Autodesk Fusion 360 part; units mm, degrees
(part 2 of 2)
  spline S276 degree 3 poles (42.600211, -33.226398) (42.604396, -33.231183) (42.608576, -33.235966) (42.612753, -33.240748) (43.093705, -33.791283) (43.530619, -34.323345) (43.918051, -34.838169) knots 0.77492411 0.77492411 0.77492411 0.77492411 0.7768622 0.7768622 0.7768622 1 1 1 1
  spline S277 degree 3 poles (43.918052, -34.838171) (45.010703, -36.290103) (45.798661, -37.579973) (46.316835, -38.956798) (46.437001, -39.276088) (46.541754, -39.597353) (46.632029, -39.919515) knots 0 0 0 0 0.81175235 0.81175235 0.81175235 1 1 1 1
  spline S278 degree 3 poles (46.63203, -39.919519) (46.773514, -40.424429) (46.814784, -40.814498) (46.845813, -41.227728) (46.878851, -41.667711) (46.885019, -42.098557) (46.850272, -42.55527) (46.832546, -42.788246) (46.806855, -43.024869) (46.741299, -43.319536) knots 0 0 0 0 0.38345336 0.38345336 0.38345336 0.79173139 0.79173139 0.79173139 1 1 1 1
  spline S279 degree 3 poles (46.741298, -43.319538) (46.404824, -44.831925) (45.478625, -46.0885) (44.311418, -46.957085) (43.806848, -47.332564) (43.253471, -47.641935) (42.664194, -47.885356) (42.664186, -47.885359) (42.664178, -47.885362) (42.664169, -47.885366) knots 0 0 0 0 0.69818353 0.69818353 0.69818353 1 1 1 1.00000633 1.00000633 1.00000633 1.00000633
  spline S280 degree 3 poles (42.664169, -47.885366) (42.034603, -48.145423) (41.279666, -48.346865) (40.565134, -48.400804) (40.346501, -48.417308) (40.13384, -48.423259) (39.924784, -48.422856) knots 0.00000234 0.00000234 0.00000234 0.00000234 0.76570861 0.76570861 0.76570861 1 1 1 1
  spline S281 degree 3 poles (39.924784, -48.422856) (38.818758, -48.420726) (37.665899, -48.16086) (36.622794, -47.69055) (36.179983, -47.490897) (35.751024, -47.258415) (35.321071, -46.997419) knots 0.00000396 0.00000396 0.00000396 0.00000396 0.70199531 0.70199531 0.70199531 1 1 1 1
  spline S282 degree 3 poles (35.321066, -46.997417) (34.424977, -46.45346) (33.574896, -45.800862) (32.774528, -45.054803) knots 0 0 0 0 0.31676612 0.31676612 0.31676612 0.31676612
extrude "Extrude1" add sketch "Sketch1" against normal blind 2 contours S0 S1 S2 S3 S4 S5 S6 S7 S8 S9 S10 S11 S12 S13 S14 S15 S16 S17 S18 S19 S20 S21 S22 S23 S24 S25 S26 S27 S28 S29 S30 S31 S32 S33 S34 S35 S36 S37 S38 S39 S40 S41 S42 S43 S44 S45 S46 S47 S48 S49 S50 S51 S52 S53 S54 S55 S56 S57 S58 S59 S60 S61 S62 S63 S64 S65 S66 S67 S68 S69 S70 S71 | S194 S195 S196 S197 S198 S199 S200 S201 S202 S203 S204 S205 S206 S207 S208 S209 S210 S211 S212 S213 S214 S215 S216 S217 S218 S219 S220 S221 S222 S223 S224 S225 S226 S227 S228 S229 S230 S231 S232 S233 S234 S235 S236 S237 S238 S239 S240 S241 L6 picked at (21.955896, -33.700003) picked at (39.308943, -18.601274)
extrude "Extrude2" add sketch "Sketch1" along normal blind 5 contours S0 S1 S2 S3 S4 S5 S6 S7 S8 S9 S10 S11 S12 S13 S14 S15 S16 S17 S18 S19 S20 S21 S22 S23 S24 S25 S26 S27 S28 S29 S30 S31 S32 S33 S34 S35 S36 S37 S38 S39 S40 S41 S42 S43 S44 S45 S46 S47 S48 S49 S50 S51 S52 S53 S54 S55 S56 S57 S58 S59 S60 S61 S62 S63 S64 S65 S66 S67 S68 S69 S70 S71 picked at (21.955896, -33.700003)
extrude "Extrude3" add sketch "Sketch1" along normal blind 10 contours S194 S195 S196 S197 S198 S199 S200 S201 S202 S203 S204 S205 S206 S207 S208 S209 S210 S211 S212 S213 S214 S215 S216 S217 S218 S219 S220 S221 S222 S223 S224 S225 S226 S227 S228 S229 S230 S231 S232 S233 S234 S235 S236 S237 S238 S239 S240 S241 L6 picked at (39.308943, -18.601274)
sketch "Sketch2" plane through (0, 0, 10) normal (0, 0, 1) x (-1, 0, 0)
  spline S0 degree 3 poles (-28.777152, 47.61447) (-28.158581, 48.54117) (-27.313864, 49.174865) (-26.365085, 49.423963) knots 0 0 0 0 1 1 1 1
  spline S1 degree 3 poles (-26.365085, 49.423963) (-25.870005, 49.553947) (-24.933082, 49.586358) (-24.398238, 49.491999) knots 0 0 0 0 1 1 1 1
  spline S2 degree 3 poles (-24.398238, 49.491999) (-21.853797, 49.043086) (-20.145962, 46.595318) (-19.808691, 42.913987) knots 0 0 0 0 1 1 1 1
  spline S3 degree 3 poles (-19.808691, 42.913987) (-19.738303, 42.145705) (-19.777142, 40.404034) (-19.883263, 39.569933) knots 0 0 0 0 1 1 1 1
  spline S4 degree 3 poles (-19.883263, 39.569933) (-19.974868, 38.849932) (-20.169101, 37.728624) (-20.298509, 37.172733) knots 0 0 0 0 1 1 1 1
  spline S5 degree 3 poles (-20.298509, 37.172733) (-20.350138, 36.950954) (-20.383684, 36.760803) (-20.373056, 36.750176) knots 0 0 0 0 1 1 1 1
  spline S6 degree 3 poles (-20.373056, 36.750176) (-20.362429, 36.739548) (-20.207496, 36.975057) (-20.02876, 37.273529) knots 0 0 0 0 1 1 1 1
  spline S7 degree 3 poles (-20.02876, 37.273529) (-18.11849, 40.463515) (-15.8391, 43.11864) (-13.903666, 44.40829) knots 0 0 0 0 1 1 1 1
  spline S8 degree 3 poles (-13.903666, 44.40829) (-13.13197, 44.9225) (-12.4509, 45.23528) (-11.669465, 45.434349) knots 0 0 0 0 1 1 1 1
  spline S9 degree 3 poles (-11.669465, 45.434349) (-11.12034, 45.574233) (-10.211189, 45.587693) (-9.705467, 45.463417) knots 0 0 0 0 1 1 1 1
  spline S10 degree 3 poles (-9.705467, 45.463417) (-8.958562, 45.27987) (-8.179688, 44.834118) (-7.596024, 44.256169) knots 0 0 0 0 1 1 1 1
  spline S11 degree 3 poles (-7.596024, 44.256169) (-6.902032, 43.568975) (-6.551135, 42.561718) (-6.474, 41.035376) knots 0 0 0 0 1 1 1 1
  spline S12 degree 3 poles (-6.474, 41.035376) (-6.338825, 38.360532) (-7.582333, 35.682392) (-10.063361, 33.304973) knots 0 0 0 0 1 1 1 1
  spline S13 degree 3 poles (-10.063361, 33.304973) (-10.912309, 32.49148) (-11.717344, 31.841911) (-12.942719, 30.981678) knots 0 0 0 0 1 1 1 1
  spline S14 degree 3 poles (-12.942719, 30.981678) (-13.486476, 30.599953) (-14.664879, 29.844231) (-14.781144, 29.80268) knots 0 0 0 0 1 1 1 1
  spline S15 degree 3 poles (-14.781144, 29.80268) (-14.813838, 29.790993) (-14.829778, 29.770067) (-14.816565, 29.756169) knots 0 0 0 0 1 1 1 1
  spline S16 degree 3 poles (-14.816565, 29.756169) (-14.803352, 29.742275) (-14.554706, 29.781213) (-14.264021, 29.842704) knots 0 0 0 0 1 1 1 1
  spline S17 degree 3 poles (-14.264021, 29.842704) (-13.428167, 30.019514) (-12.387035, 30.189924) (-11.439225, 30.305062) knots 0 0 0 0 1 1 1 1
  spline S18 degree 3 poles (-11.439225, 30.305062) (-10.694335, 30.39555) (-10.318137, 30.411456) (-8.906743, 30.412145) knots 0 0 0 0 1 1 1 1
  spline S19 degree 3 poles (-8.906743, 30.412145) (-7.429716, 30.412867) (-7.176998, 30.401447) (-6.587244, 30.307359) knots 0 0 0 0 1 1 1 1
  spline S20 degree 3 poles (-6.587244, 30.307359) (-4.61966, 29.993447) (-3.257425, 29.398503) (-2.302777, 28.436158) knots 0 0 0 0 1 1 1 1
  spline S21 degree 3 poles (-2.302777, 28.436158) (-1.404569, 27.53071) (-0.964594, 26.480042) (-0.898892, 25.083663) knots 0 0 0 0 1 1 1 1
  spline S22 degree 3 poles (-0.898892, 25.083663) (-0.752423, 21.97074) (-2.495588, 19.901678) (-5.951833, 19.086041) knots 0 0 0 0 1 1 1 1
  spline S23 degree 3 poles (-5.951833, 19.086041) (-8.285184, 18.535394) (-11.801198, 18.57942) (-15.197135, 19.201807) knots 0 0 0 0 1 1 1 1
  spline S24 degree 3 poles (-15.197135, 19.201807) (-15.472515, 19.252277) (-15.706188, 19.285206) (-15.71641, 19.274984) knots 0 0 0 0 1 1 1 1
  spline S25 degree 3 poles (-15.71641, 19.274984) (-15.726633, 19.264761) (-15.663483, 19.206281) (-15.576077, 19.145026) knots 0 0 0 0 1 1 1 1
  spline S26 degree 3 poles (-15.576077, 19.145026) (-15.173173, 18.862672) (-14.403009, 18.229035) (-13.855618, 17.729554) knots 0 0 0 0 1 1 1 1
  spline S27 degree 3 poles (-13.855618, 17.729554) (-11.319411, 15.415325) (-9.535422, 12.521165) (-8.985416, 9.828637) knots 0 0 0 0 1 1 1 1
  spline S28 degree 3 poles (-8.985416, 9.828637) (-8.541535, 7.655641) (-8.849932, 5.515577) (-9.799961, 4.176243) knots 0 0 0 0 1 1 1 1
  spline S29 degree 3 poles (-9.799961, 4.176243) (-10.248531, 3.543857) (-11.043643, 3.01215) (-11.885678, 2.781482) knots 0 0 0 0 1 1 1 1
  spline S30 degree 3 poles (-11.885678, 2.781482) (-12.362987, 2.650728) (-13.37267, 2.662599) (-13.879642, 2.804928) knots 0 0 0 0 1 1 1 1
  spline S31 degree 3 poles (-13.879642, 2.804928) (-16.035873, 3.410271) (-18.317612, 5.96279) (-20.405058, 10.10473) knots 0 0 0 0 1 1 1 1
  spline S32 degree 3 poles (-20.405058, 10.10473) (-20.621428, 10.534053) (-20.809268, 10.885434) (-20.822481, 10.885577) knots 0 0 0 0 1 1 1 1
  spline S33 degree 3 poles (-20.822481, 10.885577) (-20.835694, 10.88572) (-20.839472, 10.577696) (-20.830878, 10.201083) knots 0 0 0 0 1 1 1 1
  spline S34 degree 3 poles (-20.830878, 10.201083) (-20.800341, 8.862913) (-20.965717, 7.099114) (-21.2307, 5.936803) knots 0 0 0 0 1 1 1 1
  spline S35 degree 3 poles (-21.2307, 5.936803) (-21.953131, 2.767962) (-23.46365, 0.994904) (-25.819403, 0.550548) knots 0 0 0 0 1 1 1 1
  spline S36 degree 3 poles (-25.819403, 0.550548) (-26.276354, 0.464355) (-27.303759, 0.478399) (-27.762296, 0.577105) knots 0 0 0 0 1 1 1 1
  spline S37 degree 3 poles (-27.762296, 0.577105) (-29.380756, 0.925504) (-30.471677, 2.110585) (-30.979854, 4.072385) knots 0 0 0 0 1 1 1 1
  spline S38 degree 3 poles (-30.979854, 4.072385) (-31.228572, 5.032546) (-31.272789, 5.499233) (-31.272596, 7.162009) knots 0 0 0 0 1 1 1 1
  spline S39 degree 3 poles (-31.272596, 7.162009) (-31.272402, 8.704189) (-31.219619, 9.467197) (-31.030104, 10.666355) knots 0 0 0 0 1 1 1 1
  spline S40 degree 3 poles (-31.030104, 10.666355) (-30.971872, 11.03482) (-30.969098, 11.198786) (-31.022394, 11.12191) knots 0 0 0 0 1 1 1 1
  spline S41 degree 3 poles (-31.022394, 11.12191) (-31.030028, 11.1109) (-31.140908, 10.92892) (-31.268795, 10.717512) knots 0 0 0 0 1 1 1 1
  spline S42 degree 3 poles (-31.268795, 10.717512) (-32.09923, 9.344737) (-33.682992, 7.788682) (-35.140585, 6.913456) knots 0 0 0 0 1 1 1 1
  spline S43 degree 3 poles (-35.140585, 6.913456) (-36.521936, 6.084012) (-37.649445, 5.70804) (-38.888276, 5.663775) knots 0 0 0 0 1 1 1 1
  spline S44 degree 3 poles (-38.888276, 5.663775) (-39.709456, 5.634433) (-40.245182, 5.722796) (-40.924003, 5.999548) knots 0 0 0 0 1 1 1 1
  spline S45 degree 3 poles (-40.924003, 5.999548) (-42.412514, 6.606408) (-43.266225, 7.780936) (-43.456796, 9.48414) knots 0 0 0 0 1 1 1 1
  spline S46 degree 3 poles (-43.456796, 9.48414) (-43.616225, 10.909023) (-42.996088, 13.033743) (-41.979428, 14.545917) knots 0 0 0 0 1 1 1 1
  spline S47 degree 3 poles (-41.979428, 14.545917) (-41.293675, 15.565904) (-40.264162, 16.673275) (-39.248628, 17.483241) knots 0 0 0 0 1 1 1 1
  spline S48 degree 3 poles (-39.248628, 17.483241) (-38.697195, 17.92305) (-37.559702, 18.70613) (-37.002416, 19.02959) knots 0 0 0 0 1 1 1 1
  spline S49 degree 3 poles (-37.002416, 19.02959) (-36.824039, 19.133123) (-36.678096, 19.236237) (-36.678096, 19.258731) knots 0 0 0 0 1 1 1 1
  spline S50 degree 3 poles (-36.678096, 19.258731) (-36.678096, 19.281227) (-36.695612, 19.288805) (-36.717023, 19.275573) knots 0 0 0 0 1 1 1 1
  spline S51 degree 3 poles (-36.717023, 19.275573) (-36.738434, 19.262341) (-37.173133, 19.217823) (-37.68302, 19.176643) knots 0 0 0 0 1 1 1 1
  spline S52 degree 3 poles (-37.68302, 19.176643) (-42.00013, 18.827983) (-45.508277, 19.629245) (-47.812293, 21.490171) knots 0 0 0 0 1 1 1 1
  spline S53 degree 3 poles (-47.812293, 21.490171) (-48.837616, 22.318308) (-49.53917, 23.300587) (-49.803184, 24.277686) knots 0 0 0 0 1 1 1 1
  spline S54 degree 3 poles (-49.803184, 24.277686) (-49.942622, 24.793725) (-49.943332, 25.611328) (-49.80482, 26.123575) knots 0 0 0 0 1 1 1 1
  spline S55 degree 3 poles (-49.80482, 26.123575) (-49.3646, 27.751308) (-47.772047, 29.18037) (-45.585744, 29.909516) knots 0 0 0 0 1 1 1 1
  spline S56 degree 3 poles (-45.585744, 29.909516) (-44.371551, 30.314458) (-43.211242, 30.465773) (-41.609147, 30.428102) knots 0 0 0 0 1 1 1 1
  spline S57 degree 3 poles (-41.609147, 30.428102) (-40.042242, 30.391257) (-38.585558, 30.162583) (-36.798241, 29.672875) knots 0 0 0 0 1 1 1 1
  spline S58 degree 3 poles (-36.798241, 29.672875) (-36.104288, 29.482739) (-34.502045, 28.970831) (-34.011496, 28.782527) knots 0 0 0 0 1 1 1 1
  spline S59 degree 3 poles (-34.011496, 28.782527) (-33.926302, 28.749826) (-33.923577, 28.753712) (-33.987472, 28.816798) knots 0 0 0 0 1 1 1 1
  spline S60 degree 3 poles (-33.987472, 28.816798) (-34.027112, 28.855936) (-34.286566, 29.080518) (-34.56404, 29.315872) knots 0 0 0 0 1 1 1 1
  spline S61 degree 3 poles (-34.56404, 29.315872) (-37.459824, 31.772092) (-40.176255, 34.522567) (-41.680793, 36.521819) knots 0 0 0 0 1 1 1 1
  spline S62 degree 3 poles (-41.680793, 36.521819) (-42.91714, 38.164698) (-43.5687, 39.364673) (-43.935882, 40.675021) knots 0 0 0 0 1 1 1 1
  spline S63 degree 3 poles (-43.935882, 40.675021) (-44.082376, 41.197812) (-44.118476, 42.215448) (-44.008123, 42.711464) knots 0 0 0 0 1 1 1 1
  spline S64 degree 3 poles (-44.008123, 42.711464) (-43.761857, 43.818382) (-42.875081, 44.768754) (-41.595179, 45.297459) knots 0 0 0 0 1 1 1 1
  spline S65 degree 3 poles (-41.595179, 45.297459) (-41.00791, 45.540045) (-40.577769, 45.62411) (-39.930185, 45.622861) knots 0 0 0 0 1 1 1 1
  spline S66 degree 3 poles (-39.930185, 45.622861) (-38.88069, 45.620843) (-37.959139, 45.323304) (-36.774015, 44.603896) knots 0 0 0 0 1 1 1 1
  spline S67 degree 3 poles (-36.774015, 44.603896) (-34.502488, 43.225002) (-32.467553, 40.903967) (-30.578279, 37.537086) knots 0 0 0 0 1 1 1 1
  spline S68 degree 3 poles (-30.578279, 37.537086) (-30.492135, 37.383568) (-30.414524, 37.265095) (-30.405808, 37.273811) knots 0 0 0 0 1 1 1 1
  spline S69 degree 3 poles (-30.405808, 37.273811) (-30.397093, 37.282526) (-30.409562, 37.559482) (-30.433518, 37.889264) knots 0 0 0 0 1 1 1 1
  spline S70 degree 3 poles (-30.433518, 37.889264) (-30.457475, 38.219047) (-30.477736, 39.033089) (-30.478545, 39.698245) knots 0 0 0 0 1 1 1 1
  spline S71 degree 3 poles (-30.478545, 39.698245) (-30.482926, 43.298639) (-29.92491, 45.894977) (-28.777152, 47.61447) knots 0 0 0 0 1 1 1 1
  spline S72 degree 3 poles (-32.472573, 7.085931) (-32.472337, 6.758703) (-32.47025, 6.47465) (-32.464816, 6.218515) (-32.443264, 5.202689) (-32.348926, 4.572177) (-32.141514, 3.771474) knots -0.98475985 -0.98475985 -0.98475985 -0.98475985 -0.78645882 -0.78645882 -0.78645882 -0.00000048 -0.00000048 -0.00000048 -0.00000048
  spline S73 degree 3 poles (-32.141514, 3.771474) (-31.941823, 3.000576) (-31.656083, 2.30244) (-31.269202, 1.691236) (-30.525995, 0.5171) (-29.367827, -0.304768) (-28.01483, -0.596021) knots -1 -1 -1 -1 -0.65765407 -0.65765407 -0.65765407 0 0 0 0
  spline S74 degree 3 poles (-28.014829, -0.596022) (-27.950904, -0.609782) (-27.889104, -0.620859) (-27.827195, -0.63056) (-27.463404, -0.687562) (-27.071573, -0.706087) (-26.675131, -0.706342) (-26.298777, -0.706584) (-25.956294, -0.696435) (-25.596974, -0.628658) knots -1 -1 -1 -1 -0.91970835 -0.91970835 -0.91970835 -0.44790095 -0.44790095 -0.44790095 0 0 0 0
  spline S75 degree 3 poles (-25.596974, -0.628658) (-24.497154, -0.421203) (-23.49334, 0.049053) (-22.668932, 0.765695) (-21.368047, 1.896529) (-20.539039, 3.57199) (-20.060719, 5.670071) knots -1 -1 -1 -1 -0.61209687 -0.61209687 -0.61209687 0 0 0 0
  spline S76 degree 3 poles (-20.060719, 5.670071) (-19.98592, 5.998167) (-19.921486, 6.352401) (-19.865458, 6.727006) knots -1 -1 -1 -1 -0.75017991 -0.75017991 -0.75017991 -0.75017991
  spline S77 degree 3 poles (-19.865458, 6.727006) (-19.506115, 6.170373) (-19.141135, 5.65369) (-18.770183, 5.177884) (-17.363844, 3.374033) (-15.876078, 2.119017) (-14.203993, 1.649594) knots -0.7575867 -0.7575867 -0.7575867 -0.7575867 -0.59946487 -0.59946487 -0.59946487 -0.00000016 -0.00000016 -0.00000016 -0.00000016
  spline S78 degree 3 poles (-14.203993, 1.649594) (-14.154601, 1.635728) (-14.106084, 1.623554) (-14.057883, 1.612546) (-13.622212, 1.513049) (-13.179919, 1.486531) (-12.731334, 1.490683) (-12.335824, 1.494343) (-11.971813, 1.513674) (-11.568631, 1.624122) knots -1 -1 -1 -1 -0.94446886 -0.94446886 -0.94446886 -0.44254044 -0.44254044 -0.44254044 0 0 0 0
  spline S79 degree 3 poles (-11.56863, 1.624122) (-11.508701, 1.640539) (-11.449191, 1.658047) (-11.39012, 1.676601) (-10.355489, 2.00156) (-9.438052, 2.612334) (-8.821191, 3.481973) knots -1 -1 -1 -1 -0.9459899 -0.9459899 -0.9459899 0 0 0 0
  spline S80 degree 3 poles (-8.821191, 3.481973) (-8.647751, 3.726486) (-8.494712, 3.986098) (-8.360502, 4.257492) (-7.544378, 5.907835) (-7.383214, 7.980989) (-7.809695, 10.068803) knots -1 -1 -1 -1 -0.85877638 -0.85877638 -0.85877638 -0.00000001 -0.00000001 -0.00000001 -0.00000001
  spline S81 degree 3 poles (-7.809695, 10.068803) (-8.344019, 12.684563) (-9.857007, 15.321979) (-11.995177, 17.583099) knots -1 -1 -1 -1 -0.135529 -0.135529 -0.135529 -0.135529
  spline S82 degree 3 poles (-11.995177, 17.583099) (-9.651698, 17.410094) (-7.441319, 17.501575) (-5.676216, 17.918121) knots -0.67640459 -0.67640459 -0.67640459 -0.67640459 -0.00000003 -0.00000003 -0.00000003 -0.00000003
  spline S83 degree 3 poles (-5.676216, 17.918121) (-3.741213, 18.374762) (-2.16329, 19.223358) (-1.107088, 20.50976) (-0.083649, 21.756259) (0.382779, 23.376118) (0.299782, 25.140063) knots -1 -1 -1 -1 -0.49212315 -0.49212315 -0.49212315 -0.00000001 -0.00000001 -0.00000001 -0.00000001
  spline S84 degree 3 poles (0.299782, 25.140063) (0.288429, 25.381356) (0.267255, 25.617741) (0.235266, 25.849544) (0.052564, 27.173435) (-0.525731, 28.348698) (-1.450848, 29.281272) knots -1 -1 -1 -1 -0.85099689 -0.85099689 -0.85099689 -0.00000029 -0.00000029 -0.00000029 -0.00000029
  spline S85 degree 3 poles (-1.450848, 29.281272) (-1.547282, 29.378484) (-1.647099, 29.472688) (-1.750221, 29.563762) (-2.911566, 30.58943) (-4.455271, 31.182396) (-6.398185, 31.492372) knots -1 -1 -1 -1 -0.91844647 -0.91844647 -0.91844647 0 0 0 0
  spline S86 degree 3 poles (-6.398188, 31.492372) (-6.5613, 31.518395) (-6.714675, 31.54079) (-6.878045, 31.558344) (-7.343172, 31.608321) (-7.809609, 31.612681) (-8.907329, 31.612145) knots -1 -1 -1 -1 -0.7400635 -0.7400635 -0.7400635 -0.00000004 -0.00000004 -0.00000004 -0.00000004
  spline S87 degree 3 poles (-8.907329, 31.612145) (-9.081721, 31.61206) (-9.240949, 31.611744) (-9.387832, 31.611081) (-9.687499, 31.609728) (-9.933711, 31.607004) (-10.15681, 31.601569) knots -1 -1 -1 -1 -0.87721557 -0.87721557 -0.87721557 -0.62671458 -0.62671458 -0.62671458 -0.62671458
  spline S88 degree 3 poles (-10.15681, 31.601569) (-9.84093, 31.871196) (-9.537673, 32.14671) (-9.233118, 32.438546) knots -0.34136527 -0.34136527 -0.34136527 -0.34136527 0 0 0 0
  spline S89 degree 3 poles (-9.233117, 32.438547) (-8.974453, 32.686409) (-8.727402, 32.938203) (-8.492197, 33.193771) (-6.307323, 35.5678) (-5.134749, 38.310175) (-5.275529, 41.095942) knots -1 -1 -1 -1 -0.90281087 -0.90281087 -0.90281087 0 0 0 0
  spline S90 degree 3 poles (-5.275529, 41.095942) (-5.29661, 41.513089) (-5.336609, 41.90565) (-5.399734, 42.278186) (-5.591289, 43.408642) (-6.024456, 44.38876) (-6.751681, 45.108861) knots -1 -1 -1 -1 -0.7521372 -0.7521372 -0.7521372 -0.00000071 -0.00000071 -0.00000071 -0.00000071
  spline S91 degree 3 poles (-6.751681, 45.108861) (-7.495413, 45.845312) (-8.422699, 46.383888) (-9.419095, 46.628745) knots -1 -1 -1 -1 0 0 0 0
  spline S92 degree 3 poles (-9.419098, 46.628746) (-9.682541, 46.693485) (-9.93614, 46.722202) (-10.200068, 46.73762) (-10.786586, 46.771883) (-11.387538, 46.74449) (-11.965692, 46.597212) knots -1 -1 -1 -1 -0.68965977 -0.68965977 -0.68965977 0 0 0 0
  spline S93 degree 3 poles (-11.965701, 46.597209) (-12.87689, 46.365086) (-13.713118, 45.977261) (-14.569077, 45.406903) knots -1 -1 -1 -1 -0.00000026 -0.00000026 -0.00000026 -0.00000026
  spline S94 degree 3 poles (-14.569077, 45.406903) (-14.911886, 45.178477) (-15.254546, 44.919092) (-15.598078, 44.631736) (-16.591639, 43.800646) (-17.596183, 42.734487) (-18.575476, 41.49903) knots -1 -1 -1 -1 -0.84460942 -0.84460942 -0.84460942 -0.39518925 -0.39518925 -0.39518925 -0.39518925
  spline S95 degree 3 poles (-18.575476, 41.49903) (-18.567986, 42.065666) (-18.574975, 42.600839) (-18.613695, 43.023469) knots -0.43466848 -0.43466848 -0.43466848 -0.43466848 -0.00000013 -0.00000013 -0.00000013 -0.00000013
  spline S96 degree 3 poles (-18.613695, 43.023469) (-18.792964, 44.980199) (-19.328589, 46.680005) (-20.231405, 48.014131) (-21.174019, 49.407066) (-22.560867, 50.386367) (-24.189744, 50.673748) knots -1 -1 -1 -1 -0.51078259 -0.51078259 -0.51078259 0 0 0 0
  spline S97 degree 3 poles (-24.189751, 50.673749) (-24.546559, 50.736698) (-24.905035, 50.750906) (-25.276254, 50.745394) (-25.755317, 50.73828) (-26.214933, 50.704056) (-26.669813, 50.584627) knots -1 -1 -1 -1 -0.56341737 -0.56341737 -0.56341737 -0.0000016 -0.0000016 -0.0000016 -0.0000016
  spline S98 degree 3 poles (-26.669813, 50.584627) (-27.932868, 50.253016) (-29.016834, 49.416859) (-29.775229, 48.280685) knots -1 -1 -1 -1 0 0 0 0
  spline S99 degree 3 poles (-29.77523, 48.280684) (-29.847265, 48.172766) (-29.917006, 48.062423) (-29.984476, 47.949714) (-30.98906, 46.27158) (-31.494286, 44.103071) (-31.637272, 41.383046) knots -1 -1 -1 -1 -0.94694366 -0.94694366 -0.94694366 -0.15697726 -0.15697726 -0.15697726 -0.15697726
  spline S100 degree 3 poles (-31.637272, 41.383046) (-33.018363, 43.215897) (-34.509624, 44.633123) (-36.151323, 45.629691) knots -0.65396261 -0.65396261 -0.65396261 -0.65396261 0 0 0 0
  spline S101 degree 3 poles (-36.151325, 45.629692) (-36.316378, 45.729885) (-36.478865, 45.82388) (-36.63982, 45.911774) (-37.742242, 46.513782) (-38.815354, 46.820718) (-39.92787, 46.822859) knots -1 -1 -1 -1 -0.87259897 -0.87259897 -0.87259897 -0.0000021 -0.0000021 -0.0000021 -0.0000021
  spline S102 degree 3 poles (-39.92787, 46.822859) (-40.680329, 46.82431) (-41.365365, 46.690737) (-42.05332, 46.406561) knots -1 -1 -1 -1 0 0 0 0
  spline S103 degree 3 poles (-42.053328, 46.406558) (-42.161651, 46.361811) (-42.268086, 46.314431) (-42.372532, 46.264469) (-43.780089, 45.591165) (-44.856208, 44.42513) (-45.179484, 42.972067) knots -1 -1 -1 -1 -0.93092246 -0.93092246 -0.93092246 0 0 0 0
  spline S104 degree 3 poles (-45.179484, 42.972066) (-45.269477, 42.567564) (-45.279189, 42.190068) (-45.270967, 41.782869) (-45.261103, 41.294339) (-45.223275, 40.821945) (-45.091374, 40.351235) knots -1 -1 -1 -1 -0.54539945 -0.54539945 -0.54539945 0 0 0 0
  spline S105 degree 3 poles (-45.091374, 40.351233) (-44.676032, 38.869017) (-43.922977, 37.505603) (-42.639618, 35.800255) knots -1 -1 -1 -1 0 0 0 0
  spline S106 degree 3 poles (-42.639617, 35.800255) (-41.642718, 34.475561) (-40.206304, 32.912548) (-38.553365, 31.312101) knots -1 -1 -1 -1 -0.37843695 -0.37843695 -0.37843695 -0.37843695
  spline S107 degree 3 poles (-38.553365, 31.312101) (-39.584175, 31.503217) (-40.567212, 31.603933) (-41.580937, 31.62777) knots -0.60844734 -0.60844734 -0.60844734 -0.60844734 0 0 0 0
  spline S108 degree 3 poles (-41.580938, 31.62777) (-43.272142, 31.667537) (-44.618653, 31.497025) (-45.965395, 31.047877) knots -1 -1 -1 -1 -0.00000011 -0.00000011 -0.00000011 -0.00000011
  spline S109 degree 3 poles (-45.965395, 31.047877) (-46.561441, 30.849092) (-47.122818, 30.602856) (-47.641897, 30.314192) (-49.271077, 29.40819) (-50.519992, 28.075651) (-50.963204, 26.436861) (-50.963206, 26.436851) (-50.963209, 26.436842) (-50.963211, 26.436833) knots -1 -1 -1 -1 -0.75837207 -0.75837207 -0.75837207 0 0 0 0.00000564 0.00000564 0.00000564 0.00000564
  spline S110 degree 3 poles (-50.963211, 26.436833) (-50.963214, 26.436824) (-50.963216, 26.436815) (-50.963219, 26.436805) (-51.02331, 26.214573) (-51.058271, 25.996182) (-51.080545, 25.773981) (-51.140844, 25.172463) (-51.124068, 24.565794) (-50.96164, 23.964669) knots -1.00001792 -1.00001792 -1.00001792 -1.00001792 -1 -1 -1 -0.73024687 -0.73024687 -0.73024687 -0.0000028 -0.0000028 -0.0000028 -0.0000028
  spline S111 degree 3 poles (-50.96164, 23.964669) (-50.610818, 22.666298) (-49.744301, 21.508098) (-48.566295, 20.556639) knots -1 -1 -1 -1 -0.00000047 -0.00000047 -0.00000047 -0.00000047
  spline S112 degree 3 poles (-48.566295, 20.556639) (-48.351181, 20.382895) (-48.127628, 20.217821) (-47.896164, 20.061461) (-45.945261, 18.743579) (-43.45697, 18.048348) (-40.590265, 17.91902) knots -1 -1 -1 -1 -0.91840095 -0.91840095 -0.91840095 -0.23064134 -0.23064134 -0.23064134 -0.23064134
  spline S113 degree 3 poles (-40.590265, 17.91902) (-41.493587, 17.110225) (-42.340878, 16.15906) (-42.975284, 15.215447) knots -0.82214228 -0.82214228 -0.82214228 -0.82214228 -0.00000005 -0.00000005 -0.00000005 -0.00000005
  spline S114 degree 3 poles (-42.975284, 15.215447) (-43.40481, 14.576573) (-43.758612, 13.869203) (-44.034754, 13.142071) (-44.517866, 11.869945) (-44.784456, 10.558164) (-44.649354, 9.350705) knots -1 -1 -1 -1 -0.6362988 -0.6362988 -0.6362988 -0.00000002 -0.00000002 -0.00000002 -0.00000002
  spline S115 degree 3 poles (-44.649354, 9.350705) (-44.58109, 8.740601) (-44.438742, 8.162718) (-44.212711, 7.628784) (-43.684375, 6.380736) (-42.666561, 5.414084) (-41.377034, 4.88835) knots -1 -1 -1 -1 -0.70037073 -0.70037073 -0.70037073 0 0 0 0
  spline S116 degree 3 poles (-41.377034, 4.88835) (-40.576517, 4.561982) (-39.771138, 4.431463) (-38.845426, 4.46454) knots -1 -1 -1 -1 -0.00000004 -0.00000004 -0.00000004 -0.00000004
  spline S117 degree 3 poles (-38.845426, 4.46454) (-37.390234, 4.516536) (-36.014058, 4.989261) (-34.522843, 5.884673) knots -1 -1 -1 -1 0 0 0 0
  spline S118 degree 3 poles (-34.522842, 5.884673) (-34.302176, 6.017175) (-34.082904, 6.160913) (-33.865633, 6.314097) (-33.387025, 6.651534) (-32.917086, 7.035403) (-32.471919, 7.445993) knots -1 -1 -1 -1 -0.86761491 -0.86761491 -0.86761491 -0.57599496 -0.57599496 -0.57599496 -0.57599496
  line L0 (-32.471919, 7.445993) -> (-32.472573, 7.085931)
  line L1 (-20.26897, 9.837487) -> (-20.828289, 9.692904)
  line L2 (-31.112882, 10.10473) -> (-31.540912, 10.299221)
  line L3 (-37.573662, 18.672471) -> (-37.68302, 19.176643)
  line L4 (-35.181689, 29.179889) -> (-34.880714, 29.586257)
  line L5 (-31.326897, 38.804141) -> (-30.464712, 39.023524)
  line L6 (-19.540545, 38.064704) -> (-20.080406, 38.288495)
  line L7 (-13.929533, 29.910982) -> (-14.097665, 30.216356)
  line L8 (-14.938334, 18.655953) -> (-14.77003, 19.126671)
extrude "Extrude4" cut sketch "Sketch2" against normal up to surface (5 mm away) contours S67 S68 S69 S70 L5 | S4 S5 S6 S7 L6 | S58 S59 S60 S61 L4 | S14 S15 S16 S17 L7 | S48 S49 S50 S51 L3 | S23 S24 S25 S26 L8 | S39 S40 S41 S42 L2 | S31 S32 S33 S34 L1 picked at (-30.744168, 38.571684) picked at (-19.883237, 37.875576) picked at (-34.585742, 29.092763) picked at (-14.097073, 29.990014) picked at (-37.419699, 18.959568) picked at (-14.9685, 18.99481) picked at (-31.30753, 10.373821) picked at (-20.688075, 9.999572)
equation "CuttingHeight = 10 mm"
equation "IndentHeight = 5 mm"
equation "FlangeWidth = 4 mm"
equation "CutterWidth = 1.2 mm"
equation "FlangeThickness = 2 mm"
equation "d6 = -CutterWidth"
equation "d7 = -FlangeThickness"
equation "d9 = IndentHeight"
equation "d11 = CuttingHeight"
equation "d13 = -FlangeWidth + CutterWidth"
